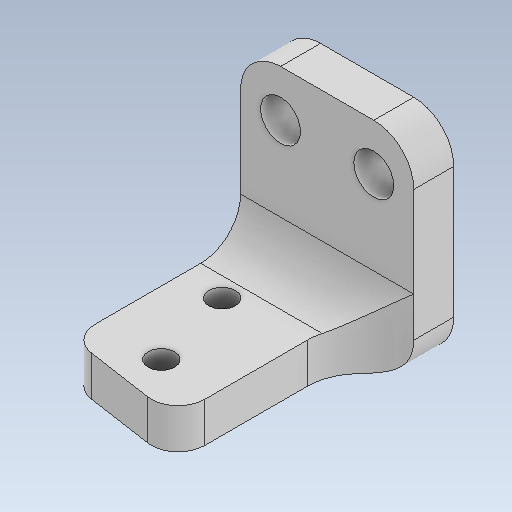
# Autodesk Inventor part: switch_holder_1
Saved by Autodesk Inventor 2020 (Build 240168000, 168)
## iProperties
Created: 2019-08-05
Part Number: switch_holder_1
Material: Generic
Document SubType Name: Modeling
Designer: psrob
Density: 1 g/cm^3
Appearance: Default
Author: psrob
Autodesk Inventor part; units mm, degrees
ref_plane "YZ Plane" through (0, 0, 0) normal (1, 0, 0) x (0, 1, 0)
ref_plane "XZ Plane" through (0, 0, 0) normal (0, 1, 0) x (-1, 0, 0)
ref_plane "XY Plane" through (0, 0, 0) normal (0, 0, 1) x (1, 0, 0)
sketch "Sketch1" plane through (0, 0, 0) normal (0, 0, 1) x (1, 0, 0)
  circle A0 centre (4.5911, -15.25) radius 1.5 projected
  circle A1 centre (11.5911, -15.25) radius 1.5 projected
  ellipse E0 centre (4.5911, 1.75) end of major axis (4.5911, 0.25) minor radius 1.5 projected
  ellipse E1 centre (11.5911, 1.75) end of major axis (11.5911, 0.25) minor radius 1.5 projected
  line L0 (4.5911, -15.25) -> (11.5911, 1.75)
  line L1 (11.5911, 1.75) -> (4.5911, 1.75)
  line L2 (4.5911, 1.75) -> (11.5911, -15.25)
  line L3 (1.0911, -18.75) -> (1.0911, 5.25)
  line L4 (1.0911, 5.25) -> (15.0911, 5.25)
  line L5 (15.0911, 5.25) -> (15.0911, -18.75)
  line L6 (15.0911, -18.75) -> (1.0911, -18.75)
  line L7 (1.0911, -18.75) -> (15.0911, 5.25) construction
  line L8 (1.0911, 5.25) -> (15.0911, -18.75) construction
  point P0 (0, 0)
  point P1 (8.0911, -6.75)
  dimension "d0" = 24
  dimension "d1" = 14
  constraints: 18 end point, 3 midpoint, 2 parallel, 1 perpendicular, 1 tangent, 1 vertical
  measures "d0" distance of L3.start L3.end
  measures "d1" distance of L3.end L4.end
extrude "Extrusion1" add sketch "Sketch1" along normal blind 3 contours E0 L1 E1 L0 L2 | L3 L4 L5 L6
thicken "Thicken1" operation add thickness 0.5 both sides no extend neighbours yes toward (1, 0, 0) faces at (1.0911, -2.75, 1)
thicken "Thicken2" operation add thickness 0.5 both sides no extend neighbours yes toward (-1, 0, 0) faces at (15.0911, -10.75, 2)
sketch "Sketch2" plane through (0, 0, 3) normal (0, 0, 1) x (1, 0, 0)
  line L0 (-11.8572, -18.7754) -> (-12.4884, -15.8632) projected
  line L1 (-11.8572, -18.7754) -> (-10.8608, -16.7323) projected
  ellipse E0 centre (-9.7787, -21.7246) end of major axis (-9.7787, -15.7246) minor radius 1.9507 (-9.7787, -15.7246) -> (-10.8608, -16.7323) ccw projected
  line L2 (-9.7787, -15.7246) -> (13.4764, -15.7246) projected
  ellipse E1 centre (13.4764, -21.7246) end of major axis (13.4764, -15.7246) minor radius 1.9507 (14.509, -16.6341) -> (13.4764, -15.7246) ccw projected
  line L3 (14.509, -16.6341) -> (15.9659, -19.43) projected
  line L4 (16.5694, -16.46) -> (15.9659, -19.43) projected
  line L5 (16.5694, -16.46) -> (14.6997, -12.8658) projected
  ellipse E2 centre (15.2167, -10.3218) end of major axis (15.2167, -13.3218) minor radius 0.9754 (14.2441, -10.55) -> (14.6997, -12.8658) ccw projected
  line L6 (14.2441, -10.55) -> (-10.6729, -10.55) projected
  ellipse E3 centre (-11.6483, -10.535) end of major axis (-11.6483, -7.535) minor radius 0.9754 (-11.1072, -13.0312) -> (-10.6729, -10.55) ccw projected
  line L7 (-11.1072, -13.0312) -> (-12.4884, -15.8632) projected
  line L8 (1.5911, 5.25) -> (1.5911, -18.75) projected
  line L9 (1.5911, -18.75) -> (14.5911, -18.75) projected
  line L10 (14.5911, -18.75) -> (14.5911, 5.25) projected
  line L11 (14.5911, 5.25) -> (1.5911, 5.25) projected
  circle A0 centre (11.5911, -15.25) radius 1.5 projected
  ellipse E4 centre (11.5911, 1.75) end of major axis (11.5911, 3.25) minor radius 1.5 projected
  circle A1 centre (4.5911, -15.25) radius 1.5 projected
  ellipse E5 centre (4.5911, 1.75) end of major axis (4.5911, 3.25) minor radius 1.5 projected
  line L12 (1.5911, 5.25) -> (1.5911, -18.75) projected
  line L13 (1.5911, -10.55) -> (10.5911, -10.55)
  line L14 (10.5911, -10.55) -> (10.5911, -7.55)
  line L15 (10.5911, -7.55) -> (1.5911, -7.55)
  line L16 (1.5911, -7.55) -> (1.5911, -10.55)
  point P0 (0, 0)
  point P1 (1.5911, -7.55)
  dimension "d8" = 9
  dimension "d9" = 3
  constraints: 8 end point, 2 parallel, 2 point on line, 1 horizontal, 1 perpendicular, 6 other
  measures "d8" distance of L15.end L14.end
  measures "d9" distance of L14.end L13.end
extrude "Extrusion2" add sketch "Sketch2" along normal blind 3 contours L8 L15 L14 L6
sketch "Sketch3" plane through (1.5911, -10.55, 3) normal (0, -1, 0) x (1, 0, 0)
  line L0 (9, 0) -> (0, 0) projected
  line L1 (9, 0) -> (9, 3) projected
  line L2 (0, 3) -> (9, 3) projected
  line L3 (0, 0) -> (0, 3) projected
  line L4 (9, 0) -> (9, 3) projected
  line L5 (9, 0) -> (-2.3137, 11.3137)
  line L6 (0, 0) -> (0, 3) projected
  line L7 (0, 0) -> (-4.2426, 4.2426)
  line L8 (-4.2426, 4.2426) -> (-2.3137, 11.3137)
  point P0 (-1.5911, -3)
  point P1 (6, 3)
  dimension "d12" = 16
  dimension "d13" = 45
  dimension "d14" = 6
  constraints: 6 end point, 1 parallel
  measures "d12" distance of L0.start L5.end
  measures "d13" angle of L0 L5
  measures "d14" distance of L0.end L7.end
extrude "Extrusion3" add sketch "Sketch3" against normal up to surface (3 mm away) contours L7 L8 L5 L2 L3
sketch "Sketch4" plane through (10.5911, -10.55, 3) normal (0, -1, 0) x (1, 0, 0)
  line L0 (0, 0) -> (-9, 0) projected
  line L1 (0, 0) -> (0, 3) projected
  line L2 (-3, 3) -> (0, 3) projected
  line L3 (-3, 3) -> (-11.3137, 11.3137) projected
  line L4 (-11.3137, 11.3137) -> (-13.2426, 4.2426) projected
  line L5 (-13.2426, 4.2426) -> (-9, 0) projected
  line L6 (0, 3) -> (-3, 3) projected
  line L7 (0, 3) -> (0, 13)
  line L8 (0, 13) -> (-11.3137, 11.3137)
  point P0 (-10.5911, -3)
  dimension "d17" = 10
  constraints: 4 end point, 1 vertical
  measures "d17" distance of L1.end L7.end
extrude "Extrusion4" add sketch "Sketch4" against normal up to surface (3 mm away) contours L2 L3 L8 L7
sketch "Sketch5" plane through (1.5911, -10.55, 3) normal (0, -1, 0) x (1, 0, 0)
  circle A0 centre (3.0722, 4.4592) radius 1 projected
  line L0 (9, 0) -> (0, 0) projected
  line L1 (9, 0) -> (9, 13) projected
  line L2 (9, 13) -> (-2.3137, 11.3137) projected
  line L3 (-2.3137, 11.3137) -> (-4.2426, 4.2426) projected
  line L4 (-4.2426, 4.2426) -> (0, 0) projected
  circle A1 centre (4.7829, 10.7301) radius 1 projected
  point P0 (-1.5911, -3)
extrude "Extrusion5" cut sketch "Sketch5" against normal blind 10 contours A0 | A1
thicken "Thicken3" operation add thickness 1 both sides no extend neighbours yes toward (-0.14742, 0, 0.989074) faces at (3.0487, -8.55, 14.8758)
sketch "Sketch6" plane through (1.5911, -7.55, 3) normal (0, 1, 0) x (1, 0, 0)
  circle A0 centre (4.7829, -10.7301) radius 1 projected
  circle A1 centre (3.0722, -4.4592) radius 1 projected
  line L0 (0, 0) -> (9, 0) projected
  line L1 (-4.2426, -4.2426) -> (0, 0) projected
  line L2 (-2.0262, -12.3676) -> (-4.2426, -4.2426) projected
  line L3 (9, -14.011) -> (-2.0262, -12.3676) projected
  line L4 (9, 0) -> (9, -14.011) projected
  line L5 (9, 0) -> (0, 0) projected
  line L6 (0, 0) -> (0, -12.6696)
  line L7 (9, -14.011) -> (-2.0262, -12.3676) projected
  point P0 (-1.5911, 3)
  constraints: 2 end point, 1 point on line, 1 vertical
extrude "Extrusion6" cut sketch "Sketch6" against normal blind 10 contours L6 L3 L2 L1
fillet "Fillet1" radius 2 2 edges at (1.5911, -9.05, 15.6696) (10.5911, -9.05, 17.011)
fillet "Fillet2" radius 4 1 edges at (10.5911, -9.05, 3)
sketch "Sketch7" plane through (0, 0, 3) normal (0, 0, 1) x (1, 0, 0)
  line L0 (14.5911, -10.55) -> (1.5911, -10.55) projected
  line L1 (1.5911, -10.55) -> (1.5911, -18.75) projected
  line L2 (1.5911, -18.75) -> (14.5911, -18.75) projected
  line L3 (14.5911, -18.75) -> (14.5911, -10.55) projected
  circle A0 centre (4.5911, -15.25) radius 1.5 projected
  circle A1 centre (11.5911, -15.25) radius 1.5 projected
  point P0 (0, 0)
extrude "Extrusion7" cut sketch "Sketch7" against normal blind 10
fillet "Fillet5" radius 3 1 edges at (8.0911, -7.55, 3)
fillet "Fillet6" radius 3 3 edges at (14.5911, 5.25, 1.5) (1.5911, 5.25, 1.5) (14.5911, -10.55, 1.5)
body "Solid1"
